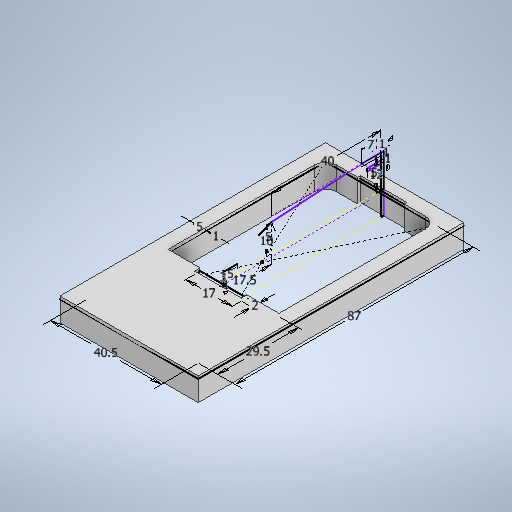
# Autodesk Inventor part: manija_puerta_marco_front_right_v3
Saved by Autodesk Inventor 2025.1 (Build 291241020, 241B)
## iProperties
Created: 2024-12-04
Part Number: manija_puerta_marco_front_right_v3
Material: Genérico
Document SubType Name: Modeling
Designer: ctamashiro
Density: 1 g/cm^3
Appearance: Valor por defecto
Author: ctamashiro
Autodesk Inventor part; units mm, degrees
ref_plane "YZ Plane" through (0, 0, 0) normal (1, 0, 0) x (0, 1, 0)
ref_plane "XZ Plane" through (0, 0, 0) normal (0, 1, 0) x (-1, 0, 0)
ref_plane "XY Plane" through (0, 0, 0) normal (0, 0, 1) x (1, 0, 0)
sketch "Boceto1" plane through (0, 0, 0) normal (0, 1, 0) x (-1, 0, 0)
  line L0 (20.25, -43.5) -> (-20.25, -43.5)
  line L1 (-20.25, -43.5) -> (-20.25, 43.5)
  line L2 (-20.25, 43.5) -> (20.25, 43.5)
  line L3 (20.25, 43.5) -> (20.25, -43.5)
  line L4 (20.25, -43.5) -> (-20.25, 43.5) construction
  line L5 (-20.25, -43.5) -> (20.25, 43.5) construction
  line L6 (25.25, -48.5) -> (-25.25, -48.5)
  line L7 (-25.25, -48.5) -> (-25.25, 48.5)
  line L8 (-25.25, 48.5) -> (25.25, 48.5)
  line L9 (25.25, 48.5) -> (25.25, -48.5)
  line L10 (20.25, 43.5) -> (-20.25, 43.5)
  line L11 (-20.25, 43.5) -> (-20.25, 14)
  line L12 (-20.25, 14) -> (20.25, 14)
  line L13 (20.25, 14) -> (20.25, 43.5)
  line L14 (25.25, 14) -> (-25.25, 14)
  line L15 (21.25, -44.5) -> (-21.25, -44.5)
  line L16 (-21.25, -44.5) -> (-21.25, 44.5)
  line L17 (-21.25, 44.5) -> (21.25, 44.5)
  line L18 (21.25, 44.5) -> (21.25, -44.5)
  line L19 (8.5, 14) -> (-8.5, 14)
  line L20 (-8.5, 14) -> (-8.5, 16)
  line L21 (-8.5, 16) -> (8.5, 16)
  line L22 (8.5, 16) -> (8.5, 14)
  point P0 (0, 0)
  point P1 (0, 0)
  point P2 (-20.25, 14)
  point P3 (-20.25, 14)
  point P4 (20.25, 14)
  point P5 (20.25, 14)
  point P6 (0, 14)
  dimension "d0" = 40.5
  dimension "d1" = 87
  dimension "d2" = 5
  dimension "d3" = 29.5
  dimension "d19" = 1
  dimension "d29" = 17
  dimension "d32" = 2
  constraints: 46 end point, 10 parallel, 6 point on line, 5 perpendicular, 4 midpoint, 3 horizontal, 1 coincident, 6 other
  measures "d0" distance of L1.end L2.end
  measures "d1" distance of L0.end L1.end
  measures "d2" distance between parallel lines of L3 L9
  measures "d3" distance of L11.end L10.end
  measures "d19" distance between parallel lines of L3 L18
  measures "d29" distance of L20.end L21.end
  measures "d32" distance between parallel lines of L21 L19
extrude "Extrusión4" add sketch "Boceto1" against normal blind 7.5 contours L3 L14 L18 L15 L16 L1 L0 | L3 L2 L1 L14 L16 L17 L18 | L18 L17 L16 L14 L7 L8 L9 | L14 L9 L6 L7 L16 L15 L18
extrude "Extrusión5" add sketch "Boceto1" along normal blind 1 contours L3 L14 L18 L15 L16 L1 L0 | L12 L22 L21 L20 L1 L2 L3 | L3 L2 L1 L14 L16 L17 L18 | L12 L20 L21 L22 | L18 L17 L16 L14 L7 L8 L9 | L14 L9 L6 L7 L16 L15 L18
fillet "Empalme2" radius 4 4 edges at (-20.25, -3.25, -43.5) (20.25, -3.25, -43.5) (20.25, -3.75, 43.5) (-20.25, -3.75, 43.5)
fillet "Empalme3" radius 2 1 edges at (0, 0, 14)
sketch "Boceto2" plane through (0, 0, 0) normal (1, 0, 0) x (0, 1, 0)
  line L0 (1, 14) -> (1, -39.5) construction
  line L1 (1, 14) -> (4, 14)
  line L2 (4, 14) -> (4, 9)
  line L3 (1, -3.5) -> (11, -3.5) construction
  line L4 (4, 14) -> (11, -3.5)
  line L5 (11, -3.5) -> (9.143, 1.1424)
  line L6 (0, 15) -> (0, -39.5) construction
  line L7 (1, -43.5) -> (1, -39.5) construction
  line L8 (1, -43.5) -> (13, -43.5)
  line L9 (13, -43.5) -> (10.5, -43.5)
  line L10 (1, -43.5) -> (13, -43.5)
  line L11 (13, -43.5) -> (13, -44.5)
  line L12 (13, -44.5) -> (1, -44.5)
  line L13 (1, -44.5) -> (1, -43.5)
  line L14 (10.5, -43.5) -> (10.5, -38.5)
  line L15 (10.5, -38.5) -> (9.5, -38.5)
  line L16 (9.5, -38.5) -> (9.5, -43.5)
  line L17 (9.5, -43.5) -> (10.5, -43.5)
  line L18 (10.5, -43.5) -> (10.5, -38.5)
  line L19 (13, -43.5) -> (13, -3.5) construction
  line L20 (13, -43.5) -> (13, -36.5) construction
  line L21 (13, -36.5) -> (12, -36.5) construction
  line L22 (13, -36.5) -> (13, -43.5)
  line L23 (11, -3.5) -> (13, -36.5)
  line L24 (1, 14) -> (-1, 14)
  line L25 (-1, 14) -> (-1, 43.5)
  line L26 (0, 43.5) -> (-7.5, 43.5) projected
  line L27 (0, 39.5) -> (0, 15.7321) projected
  line L28 (-7.5, 48.5) -> (-7.5, -48.5) construction
  line L29 (1, -43.5) -> (-7.5, -43.5)
  line L30 (-7.5, -43.5) -> (-7.5, -44.5)
  line L31 (-7.5, -44.5) -> (1, -44.5)
  line L32 (1, -44.5) -> (1, -43.5)
  point P0 (0, 0)
  dimension "d22" = 3
  dimension "d23" = 5
  dimension "d24" = 10
  dimension "d25" = 17.5
  dimension "d26" = 5
  dimension "d33" = 12
  dimension "d36" = 1
  dimension "d37" = 5
  dimension "d38" = 1
  dimension "d39" = 40
  dimension "d40" = 7
  dimension "d41" = 1
  dimension "d48" = 1
  constraints: 56 end point, 7 horizontal, 7 parallel, 7 perpendicular, 6 point on line, 1 collinear, 1 vertical
  measures "d22" distance of L0.start L1.end
  measures "d23" distance of L1.end L2.end
  measures "d24" distance of L3.start L3.end
  measures "d25" distance between parallel lines of L3 L1
  measures "d26" distance of L3.end L5.end
  measures "d33" distance of L7.start L8.end
  measures "d36" distance of L10.end L11.end
  measures "d37" distance of L9.end L14.end
  measures "d38" distance of L17.end L16.end
  measures "d39" distance of L10.end L19.end
  measures "d40" distance of L10.end L20.end
  measures "d41" distance of L20.end L21.end
  measures "d48" distance between parallel lines of L27 L25
feature "Barrido1" [suppressed]
extrude "Extrusión7" [suppressed]
extrude "Extrusión8" cut sketch "Boceto1" along normal blind 10 contours L12 L20 L21 L22
extrude "Extrusión9" cut sketch "Boceto2" along normal mid plane 17 contours L13 L31 L30 L29
